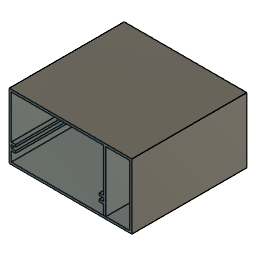
Boitier DD tube v2 (Autodesk Fusion 360 design; units mm, degrees)
part number: 2025-12-18-08-30-15-835
Autodesk Fusion 360 part; units mm, degrees
sketch "Esquisse1" plane through (0, 0, 0) normal (0, 1, 0) x (1, 0, 0)
  line L0 (0, 0) -> (-56.5, 0)
  line L1 (-56.5, 0) -> (-56.5, -30)
  line L2 (-56.5, -30) -> (0, -30)
  line L3 (0, -30) -> (0, 0)
  line L4 (-1, -29) -> (-55.5331, -29)
  line L5 (-55.5331, -29) -> (-55.5331, -1.0074)
  line L6 (-55.5331, -1.0074) -> (-1, -1.0074)
  line L7 (-1, -1.0074) -> (-1, -29)
  line L8 (-55.5331, -1.0074) -> (-1.0331, -1.0074)
  line L9 (-1.0331, -1.0074) -> (-1.0331, -28.0074)
  line L10 (-55.5331, -28.0074) -> (-55.5331, -1.0074)
  line L11 (-12, -29) -> (-13, -29)
  line L12 (-13, -29) -> (-13, -1)
  line L13 (-13, -1) -> (-12, -1)
  line L14 (-12, -1) -> (-12, -29)
  line L15 (-13, -9) -> (-15, -9)
  line L16 (-15, -9) -> (-15, -8)
  line L17 (-15, -8) -> (-13, -8)
  line L18 (-13, -8) -> (-13, -9)
  line L19 (-13, -6.485) -> (-15, -6.485)
  line L20 (-15, -6.485) -> (-15, -5.485)
  line L21 (-15, -5.485) -> (-13, -5.485)
  line L22 (-13, -5.485) -> (-13, -6.485)
  line L23 (-55.5331, -8.9771) -> (-53.5331, -8.9771)
  line L24 (-53.5331, -8.9771) -> (-53.5331, -7.9771)
  line L25 (-53.5331, -7.9771) -> (-55.5331, -7.9771)
  line L26 (-55.5331, -7.9771) -> (-55.5331, -8.9771)
  line L27 (-55.5331, -6.5064) -> (-53.5331, -6.5064)
  line L28 (-53.5331, -6.5064) -> (-53.5331, -5.5064)
  line L29 (-53.5331, -5.5064) -> (-55.5331, -5.5064)
  line L30 (-55.5331, -5.5064) -> (-55.5331, -6.5064)
  constraint horizontal L0
  constraint vertical L1
  constraint horizontal L2
  constraint vertical L3
  constraint coincident L0.start L3.end
  constraint horizontal L4
  constraint vertical L5
  constraint horizontal L6
  constraint vertical L7
  constraint horizontal L8
  constraint vertical L9
  constraint vertical L10
  constraint horizontal L11
  constraint vertical L12
  constraint horizontal L13
  constraint vertical L14
  constraint coincident L4 L11.start
  constraint horizontal L15
  constraint vertical L16
  constraint horizontal L17
  constraint vertical L18
  constraint coincident L12 L15.start
  constraint horizontal L19
  constraint vertical L20
  constraint horizontal L21
  constraint vertical L22
  constraint coincident L12 L19.start
  constraint horizontal L23
  constraint vertical L24
  constraint horizontal L25
  constraint vertical L26
  constraint coincident L5 L23.start
  constraint horizontal L27
  constraint vertical L28
  constraint horizontal L29
  constraint vertical L30
  constraint coincident L10 L27.start
extrude "Extrusion2" add sketch "Esquisse1" along normal blind 53 contours L0 L1 L2 L3 | L4 L6 L8 L11 L12 L14 L18 L22 | L12 L15 L16 L17 L18 | L12 L19 L20 L21 L22 | L5 L10 L23 L24 L25 L26 | L5 L10 L27 L28 L29 L30
sketch "Esquisse2" plane through (0, 0, 0) normal (0, -1, 0) x (1, 0, 0)
  line L0 (-12, 1.0074) -> (-12, 29)
  line L1 (-12, 29) -> (-1, 29)
  line L2 (-1, 29) -> (-1, 1.0074)
  line L3 (-1, 1.0074) -> (-12, 1.0074)
  line L4 (-12, 1.0074) -> (-12, 1)
  line L5 (-12, 1) -> (-13, 1)
  line L6 (-13, 1) -> (-13, 1.0074)
  line L7 (-13, 1.0074) -> (-55.5331, 1.0074)
  line L8 (-55.5331, 1.0074) -> (-55.5331, 5.5064)
  line L9 (-55.5331, 5.5064) -> (-53.5331, 5.5064)
  line L10 (-53.5331, 5.5064) -> (-53.5331, 6.5064)
  line L11 (-53.5331, 6.5064) -> (-55.5331, 6.5064)
  line L12 (-55.5331, 6.5064) -> (-55.5331, 7.9771)
  line L13 (-55.5331, 7.9771) -> (-53.5331, 7.9771)
  line L14 (-53.5331, 7.9771) -> (-53.5331, 8.9771)
  line L15 (-53.5331, 8.9771) -> (-55.5331, 8.9771)
  line L16 (-55.5331, 8.9771) -> (-55.5331, 29)
  line L17 (-55.5331, 29) -> (-13, 29)
  line L18 (-13, 29) -> (-13, 9)
  line L19 (-13, 9) -> (-15, 9)
  line L20 (-15, 9) -> (-15, 8)
  line L21 (-15, 8) -> (-13, 8)
  line L22 (-13, 8) -> (-13, 6.485)
  line L23 (-13, 6.485) -> (-15, 6.485)
  line L24 (-15, 6.485) -> (-15, 5.485)
  line L25 (-15, 5.485) -> (-13, 5.485)
  line L26 (-13, 5.485) -> (-13, 1.0074)
  line L27 (-13, 1.0074) -> (-12, 1.0074)
  line L28 (0, 0) -> (0, 30)
  line L29 (0, 30) -> (-56.5, 30)
  line L30 (-56.5, 30) -> (-56.5, 0)
  line L31 (-56.5, 0) -> (0, 0)
extrude "Extrusion1" [suppressed]
